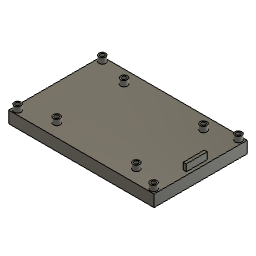
waveshare_4_3_dsi_LCD (Autodesk Fusion 360 design; units mm, degrees)
Autodesk Fusion 360 part; units mm, degrees
sketch "lcd" plane through (0, 0, 0) normal (0, 1, 0) x (1, 0, 0)
  line L0 (53, -34) -> (-53, -34)
  line L1 (-53, -34) -> (-53, 34)
  line L2 (-53, 34) -> (53, 34)
  line L3 (53, 34) -> (53, -34)
  line L4 (53, -34) -> (-53, 34) construction
  line L5 (-53, -34) -> (53, 34) construction
  line L6 (49.65, -30.9) -> (-49.65, -30.9) construction
  line L7 (-49.65, -30.9) -> (-49.65, 30.9) construction
  line L8 (-49.65, 30.9) -> (49.65, 30.9) construction
  line L9 (49.65, 30.9) -> (49.65, -30.9) construction
  line L10 (49.65, -30.9) -> (-49.65, 30.9) construction
  line L11 (-49.65, -30.9) -> (49.65, 30.9) construction
  circle A0 centre (-49.65, 30.9) radius 1.5
  circle A1 centre (-49.65, 30.9) radius 2.5
  circle A2 centre (-49.65, -30.9) radius 2.5
  circle A3 centre (-49.65, -30.9) radius 1.5
  circle A4 centre (49.65, -30.9) radius 2.5
  circle A5 centre (49.65, -30.9) radius 1.5
  circle A6 centre (49.65, 30.9) radius 2.5
  circle A7 centre (49.65, 30.9) radius 1.5
  circle A8 centre (-27.38, -24.54) radius 2.5
  circle A9 centre (-27.38, -24.54) radius 1.5
  circle A10 centre (30.62, -24.54) radius 1.5
  circle A11 centre (30.62, -24.54) radius 2.5
  circle A12 centre (-27.38, 24.5) radius 1.5
  circle A13 centre (-27.38, 24.5) radius 2.5
  circle A14 centre (30.62, 24.5) radius 2.5
  circle A15 centre (30.62, 24.5) radius 1.5
  line L12 (48.5612, 7.0715) -> (50.7124, 7.0715)
  line L13 (50.7124, 7.0715) -> (50.7124, -8.2737)
  line L14 (50.7124, -8.2737) -> (48.5612, -8.2737)
  line L15 (48.5612, -8.2737) -> (48.5612, 7.0715)
  dimension "d1" = 106
  dimension "d2" = 68
  dimension "d3" = 99.3
  dimension "d4" = 61.8
  dimension "d5" = 3
  dimension "d6" = 5
  dimension "d7" = 3
  dimension "d8" = 5
  dimension "d9" = 3
  dimension "d10" = 5
  dimension "d11" = 3
  dimension "d12" = 5
  dimension "d13" = 3
  dimension "d14" = 5
  dimension "d15" = 9.46
  dimension "d16" = 25.62
  dimension "d17" = 3
  dimension "d18" = 5
  dimension "d19" = 22.38
  dimension "d20" = 3
  dimension "d21" = 5
  dimension "d22" = 3
  dimension "d23" = 5
  dimension "d24" = 9.5
  dimension "d25" = 9.5
  constraint horizontal L0
  constraint perpendicular L0 L1
  constraint parallel L0 L2
  constraint parallel L1 L3
  constraint coincident L4 origin
  constraint coincident L5 origin
  constraint horizontal L6
  constraint perpendicular L6 L7
  constraint parallel L6 L8
  constraint parallel L7 L9
  constraint coincident L10 origin
  constraint coincident L11 origin
  constraint coincident L7.end L8.start
  constraint concentric A0 A1
  constraint concentric A2 A3
  constraint concentric A6 A7
  constraint concentric A4 A5
  constraint concentric A8 A9
  constraint concentric A10 A11
  constraint concentric A12 A13
  constraint concentric A14 A15
  constraint horizontal L12
  constraint vertical L13
  constraint horizontal L14
  constraint vertical L15
  measures "d1" distance of L1.end L2.end
  measures "d2" distance of L0.end L1.end
  measures "d3" distance of L7.end L8.end
  measures "d4" distance of L6.end L7.end
  measures "d5" diameter of A0
  measures "d6" diameter of A1
  measures "d7" diameter of A3
  measures "d8" diameter of A2
  measures "d9" diameter of A7
  measures "d10" diameter of A6
  measures "d11" diameter of A5
  measures "d12" diameter of A4
  measures "d13" diameter of A9
  measures "d14" diameter of A8
  measures "d15" distance of L0 A8.centre
  measures "d16" distance of L1 A8.centre
  measures "d17" diameter of A10
  measures "d18" diameter of A11
  measures "d19" distance of L3 A10.centre
  measures "d20" diameter of A12
  measures "d21" diameter of A13
  measures "d22" diameter of A15
  measures "d23" diameter of A14
  measures "d24" distance of L2 A12.centre
  measures "d25" distance of L2 A14.centre
extrude "Extrude1" add sketch "lcd" against normal blind 8.6 contours L0 L1 L2 L3 | A0 | A1 | A2 | A3 | A4 | A5 | A6 | A7 | A8 | A9 | A10 | A11 | A12 | A13 | A14 | A15 | L12 L13 L14 L15
extrude "Extrude2" add sketch "lcd" along normal blind 4 contours A1 | A2 | A4 | A6 | A8 | A11 | A13 | A14
extrude "Extrude3" add sketch "lcd" along normal blind 5 contours L12 L13 L14 L15
named bodies: "4.3_dsi_lcd"
